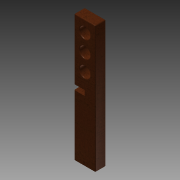
# Autodesk Inventor part: stand1
Saved by Autodesk Inventor 2015 (Build 190159000, 159)
## iProperties
Created: 2014-07-19
Part Number: stand1
Material: Wood (Walnut)
Document SubType Name: Modeling
Designer: pc
Density: 0.55 g/cm^3
Appearance: Walnut - Natural Polished
Author: pc
Autodesk Inventor part; units mm, degrees
ref_plane "YZ Plane" through (0, 0, 0) normal (1, 0, 0) x (0, 1, 0)
ref_plane "XZ Plane" through (0, 0, 0) normal (0, 1, 0) x (-1, 0, 0)
ref_plane "XY Plane" through (0, 0, 0) normal (0, 0, 1) x (1, 0, 0)
sketch "Sketch1" plane through (0, 0, 0) normal (0, 1, 0) x (-1, 0, 0)
  line L0 (25, 150) -> (-25, 150)
  line L1 (-25, 150) -> (-25, -150)
  line L2 (-25, -150) -> (25, -150)
  line L3 (25, -150) -> (25, 150)
  line L4 (25, 150) -> (-25, -150) construction
  line L5 (-25, 150) -> (25, -150) construction
  point P0 (0, 0)
  dimension "d0" = 300
  dimension "d1" = 50
  constraints: 12 end point, 2 midpoint, 2 parallel, 1 horizontal, 1 perpendicular
  measures "d0" distance of L0.end L1.end
  measures "d1" distance of L0.start L0.end
extrude "Extrusion1" add sketch "Sketch1" along normal blind 25
fillet "Fillet1" radius 2 1 edges at (25, 25, 0)
fillet "Fillet2" radius 2 1 edges at (25, 0, 0)
fillet "Fillet3" radius 2 5 edges at (-1, 25, 150) (24.4142, 24.4142, 150) (25, 12.5, 150) (24.4142, 0.5858, 150) (-1, 0, 150)
fillet "Fillet4" radius 2 5 edges at (-25, 0, -1) (-25, 0.5858, 149.4142) (-25, 12.5, 150) (-25, 24.4142, 149.4142) (-25, 25, -1)
fillet "Fillet5" radius 2 8 edges at (0, 25, -150) (-24.4142, 24.4142, -150) (-25, 12.5, -150) (-24.4142, 0.5858, -150) (0, 0, -150) (24.4142, 0.5858, -150) (25, 12.5, -150) (24.4142, 24.4142, -150)
sketch "Sketch2" plane through (0, 0, 0) normal (0, -1, 0) x (1, 0, 0)
  circle A0 centre (0, 123) radius 12.5
  circle A1 centre (0, 83) radius 12.5
  circle A2 centre (0, 43) radius 12.5
  line L0 (-23, 148) -> (23, 148) projected
  line L1 (0, 83) -> (0, 43) construction
  line L2 (0, 123) -> (0, 83) construction
  line L3 (0, 0) -> (0, 148) construction
  line L4 (-39.2491, 0) -> (23.3031, 0) construction
  line L5 (0, -6) -> (-25, -6)
  line L6 (-25, -6) -> (-25, 6)
  line L7 (-25, 6) -> (0, 6)
  line L8 (0, 6) -> (0, -6)
  line L9 (0, -6) -> (-25, 6) construction
  line L10 (-25, -6) -> (0, 6) construction
  line L11 (-25, 148) -> (-25, -148) projected
  point P0 (0, 103)
  point P1 (-11.5, 0)
  point P2 (-12.5, 0)
  dimension "d9" = 25
  dimension "d10" = 25
  dimension "d11" = 25
  dimension "d12" = 40
  dimension "d13" = 40
  dimension "d14" = 25
  dimension "d16" = 12
  constraints: 20 end point, 4 midpoint, 3 centre point, 3 point on line, 2 collinear, 2 horizontal, 2 parallel, 2 vertical, 1 coincident, 1 perpendicular
  measures "d9" diameter of A0
  measures "d10" diameter of A1
  measures "d11" diameter of A2
  measures "d12" distance of L1.start L2.start
  measures "d13" distance of A2.centre L1.start
  measures "d14" distance from line of L2.start L0
  measures "d16" distance between parallel lines of L5 L7
extrude "Extrusion3" cut sketch "Sketch2" against normal through all
fillet "Fillet6" radius 2 1 edges at (-12.5, 0, 43)
fillet "Fillet7" radius 2 1 edges at (-12.5, 0, 83)
fillet "Fillet8" radius 2 1 edges at (-12.5, 0, 123)
fillet "Fillet9" radius 2 1 edges at (-12.5, 25, 123)
fillet "Fillet10" radius 2 1 edges at (-12.5, 25, 83)
fillet "Fillet11" radius 2 1 edges at (-12.5, 25, 43)
equation "\"d13\" = d12"
body "Solid1"
